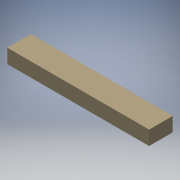
# Autodesk Inventor part: Rack and Pinion Frame Back
Saved by Autodesk Inventor 2016 (Build 200138000, 138)
## iProperties
Created: 2016-04-18
Part Number: Rack and Pinion Frame Back
Material: Generic
Document SubType Name: Modeling
Designer: Andrea
Density: 1 g/cm^3
Appearance: Wheat
Author: Andrea
Autodesk Inventor part; units mm, degrees
ref_plane "YZ Plane" through (0, 0, 0) normal (1, 0, 0) x (0, 1, 0)
ref_plane "XZ Plane" through (0, 0, 0) normal (0, 1, 0) x (-1, 0, 0)
ref_plane "XY Plane" through (0, 0, 0) normal (0, 0, 1) x (1, 0, 0)
sketch "Sketch1" plane through (0, 0, 0) normal (1, 0, 0) x (0, 1, 0)
  line L0 (-9.525, 19.05) -> (9.525, 19.05)
  line L1 (9.525, 19.05) -> (9.525, -19.05)
  line L2 (9.525, -19.05) -> (-9.525, -19.05)
  line L3 (-9.525, -19.05) -> (-9.525, 19.05)
  line L4 (-9.525, 19.05) -> (9.525, -19.05) construction
  line L5 (9.525, 19.05) -> (-9.525, -19.05) construction
  point P0 (0, 0)
  dimension "d0" = 19.05
  dimension "d1" = 38.1
  constraints: 12 end point, 2 midpoint, 2 parallel, 1 horizontal, 1 perpendicular
  measures "d0" distance of L1.end L2.end
  measures "d1" distance of L0.end L1.end
extrude "Extrusion1" add sketch "Sketch1" along normal blind 381
body "Solid1"
